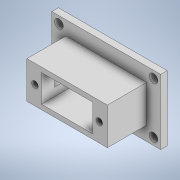
# Autodesk Inventor part: ServoESP32Base
Saved by Autodesk Inventor 2020 (Build 240168000, 168)
## iProperties
Created: 2022-11-23
Part Number: ServoESP32Base
Material: Generic
Document SubType Name: Modeling
Designer: chava4445
Density: 1 g/cm^3
Appearance: Default
Author: chava4445
Autodesk Inventor part; units mm, degrees
ref_plane "YZ Plane" through (0, 0, 0) normal (1, 0, 0) x (0, 1, 0)
ref_plane "XZ Plane" through (0, 0, 0) normal (0, 1, 0) x (-1, 0, 0)
ref_plane "XY Plane" through (0, 0, 0) normal (0, 0, 1) x (1, 0, 0)
sketch "Sketch1" plane through (0, 0, 0) normal (0, 0, 1) x (1, 0, 0)
  point P0 (0, 0)
sketch "Sketch2" plane through (0, 0, 0) normal (0, 0, 1) x (1, 0, 0)
  line L0 (-25, 15) -> (25, 15)
  line L1 (25, 15) -> (25, -15)
  line L2 (25, -15) -> (-25, -15)
  line L3 (-25, -15) -> (-25, 15)
  line L4 (-25, 15) -> (25, -15) construction
  line L5 (25, 15) -> (-25, -15) construction
  point P0 (0, 0)
  dimension "d0" = 30
  dimension "d1" = 50
  constraints: 12 end point, 2 midpoint, 2 parallel, 1 horizontal, 1 perpendicular
  measures "d0" distance of L0.end L1.end
  measures "d1" distance of L0.start L0.end
extrude "Extrusion1" add sketch "Sketch2" along normal blind 3
sketch "Sketch3" plane through (0, 0, 3) normal (0, 0, 1) x (1, 0, 0)
  line L0 (-7.2947, 3.9789) -> (7.2947, -3.9789) construction
  line L1 (7.2947, 3.9789) -> (-7.2947, -3.9789) construction
  line L2 (-11.8, 6.3) -> (11.8, 6.3)
  line L3 (11.8, 6.3) -> (11.8, -6.3)
  line L4 (11.8, -6.3) -> (-11.8, -6.3)
  line L5 (-11.8, -6.3) -> (-11.8, 6.3)
  line L6 (-11.8, 6.3) -> (11.8, -6.3) construction
  line L7 (11.8, 6.3) -> (-11.8, -6.3) construction
  line L8 (-18.5, 8.5) -> (18.5, 8.5)
  line L9 (18.5, 8.5) -> (18.5, -8.5)
  line L10 (18.5, -8.5) -> (-18.5, -8.5)
  line L11 (-18.5, -8.5) -> (-18.5, 8.5)
  line L12 (-18.5, 8.5) -> (18.5, -8.5) construction
  line L13 (18.5, 8.5) -> (-18.5, -8.5) construction
  point P0 (0, 0)
  dimension "d4" = 23.6
  dimension "d5" = 12.6
  dimension "d6" = 37
  dimension "d7" = 17
  constraints: 28 end point, 6 midpoint, 4 parallel, 2 horizontal, 2 perpendicular
  measures "d4" distance of L2.start L2.end
  measures "d5" distance of L2.end L3.end
  measures "d6" distance of L8.start L8.end
  measures "d7" distance of L8.end L9.end
extrude "Extrusion2" add sketch "Sketch3" along normal blind 18
sketch "Sketch5" plane through (-18.5, -8.5, 3) normal (-1, 0, 0) x (0, 0, 1)
  line L0 (0, 14.8) -> (0, 2.2) projected
  line L1 (0, 8.5) -> (14, 8.5) construction
  line L2 (2, 11) -> (12, 11)
  line L3 (12, 11) -> (12, 6)
  line L4 (12, 6) -> (2, 6)
  line L5 (2, 6) -> (2, 11)
  line L6 (2, 11) -> (12, 6) construction
  line L7 (12, 11) -> (2, 6) construction
  point P0 (-3, 8.5)
  point P1 (7, 8.5)
  dimension "d10" = 14
  dimension "d11" = 5
  dimension "d12" = 10
  constraints: 14 end point, 4 midpoint, 2 horizontal, 2 parallel, 1 perpendicular
  measures "d10" distance of L1.start L1.end
  measures "d11" distance of L2.end L3.end
  measures "d12" distance of L3.end L4.end
extrude "Extrusion3" cut sketch "Sketch5" against normal blind 18
sketch "Sketch6" plane through (0, 0, 21) normal (0, 0, 1) x (1, 0, 0)
  line L0 (11.8, 6.3) -> (11.8, -6.3) projected
  line L1 (11.8, 0) -> (14.8, 0) construction
  circle A0 centre (14.8, 0) radius 1.5
  line L2 (0, 0) -> (0, -10.1411) construction
  line L3 (-11.8, 0) -> (-14.8, 0) construction
  circle A1 centre (-14.8, 0) radius 1.5
  dimension "d15" = 3
  dimension "d16" = 3
  constraints: 6 end point, 3 symmetric about line, 2 centre point, 2 coincident, 1 horizontal, 1 midpoint, 1 vertical, 1 other
  measures "d15" distance of L1.start L1.end
  measures "d16" diameter of A0
extrude "Extrusion4" cut sketch "Sketch6" against normal blind 5
sketch "Sketch7" plane through (0, 0, 3) normal (0, 0, 1) x (1, 0, 0)
  point P0 (0, 0)
sketch "Sketch8" plane through (0, 0, 3) normal (0, 0, 1) x (1, 0, 0)
  line L0 (0, 0) -> (6.4971, 0) construction
  line L1 (0, 0) -> (0, -4.6086) construction
  line L2 (25, 15) -> (-25, 15) projected
  line L3 (18.5, 8.5) -> (-18.5, 8.5) projected
  line L4 (25, 15) -> (18.5, 8.5) construction
  circle A0 centre (21.75, 11.75) radius 2
  circle A1 centre (21.75, -11.75) radius 2
  circle A2 centre (-21.75, 11.75) radius 2
  circle A3 centre (-21.75, -11.75) radius 2
  dimension "d19" = 4
  constraints: 6 end point, 4 centre point, 3 symmetric about line, 1 horizontal, 1 midpoint, 1 vertical, 3 other
  measures "d19" diameter of A0
extrude "Extrusion5" cut sketch "Sketch8" against normal blind 3
body "Solid1"
